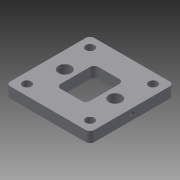
# Autodesk Inventor part: AdapterPlate
Saved by Autodesk Inventor 2015 SP1 (Build 190203100, 203)
## iProperties
Created: 2015-08-27
Part Number: AdapterPlate
Material: Generic
Document SubType Name: Modeling
Designer: I Rabey
Density: 1 g/cm^3
Appearance: Default
Author: I Rabey
Autodesk Inventor part; units mm, degrees
ref_plane "YZ Plane" through (0, 0, 0) normal (1, 0, 0) x (0, 1, 0)
ref_plane "XZ Plane" through (0, 0, 0) normal (0, 1, 0) x (-1, 0, 0)
ref_plane "XY Plane" through (0, 0, 0) normal (0, 0, 1) x (1, 0, 0)
sketch "Sketch1" plane through (0, 0, 0) normal (0, 1, 0) x (-1, 0, 0)
  line L0 (-17.5, -17.5) -> (17.5, 17.5) construction
  line L1 (17.5, -17.5) -> (-17.5, 17.5) construction
  circle A0 centre (15, -15) radius 2.05
  circle A1 centre (-15, -15) radius 2.05
  circle A2 centre (-15, 15) radius 2.05
  circle A3 centre (15, 15) radius 2.05
  line L2 (20, 20) -> (-20, 20)
  line L3 (-20, 20) -> (-20, -20)
  line L4 (-20, -20) -> (20, -20)
  line L5 (20, -20) -> (20, 20)
  line L6 (20, 20) -> (-20, -20) construction
  line L7 (-20, 20) -> (20, -20) construction
  circle A4 centre (12, 0) radius 3.05
  circle A5 centre (-12, 0) radius 3.05
  point P0 (0, 0)
  dimension "d0" = 35
  dimension "d1" = 35
  dimension "d2" = 4.1
  dimension "d3" = 4.1
  dimension "d4" = 4.1
  dimension "d5" = 4.1
  dimension "d6" = 30
  dimension "d7" = 30
  dimension "d8" = 30
  dimension "d9" = 30
  dimension "d10" = 40
  dimension "d11" = 40
  dimension "d14" = 6.1
  dimension "d15" = 8
  dimension "d16" = 6.1
  dimension "d17" = 8
  constraints: 16 end point, 6 centre point, 4 midpoint, 4 point on line, 2 parallel, 1 horizontal, 1 perpendicular
  measures "d0" distance of L1.end L0.end
  measures "d1" distance of L1.start L0.end
  measures "d2" diameter of A0
  measures "d3" diameter of A1
  measures "d4" diameter of A2
  measures "d5" diameter of A3
  measures "d6" distance of A3.centre A0.centre
  measures "d7" distance of A0.centre A1.centre
  measures "d8" distance of A2.centre A1.centre
  measures "d9" distance of A3.centre A2.centre
  measures "d10" distance of L4.end L3.end
  measures "d11" distance of L3.end L2.end
  measures "d14" diameter of A4
  measures "d15" distance from line of A4.centre L5
  measures "d16" diameter of A5
  measures "d17" distance from line of L3 A5.centre
extrude "Extrusion2" add sketch "Sketch1" along normal blind 5
sketch "Sketch2" plane through (20, 0, 20) normal (1, 0, 0) x (0, 0, -1)
  circle A0 centre (20, 2.5) radius 1
  line L0 (0, 5) -> (40, 5) projected
  point P0 (20, 0)
  dimension "d20" = 2
  dimension "d21" = 2.5
  constraints: 1 centre point
  measures "d20" diameter of A0
  measures "d21" distance from line of A0.centre L0
hole "Hole1" at (20, 2.5, 0) direction (-1, 0, 0) diameter 2 depth 8 tip angle 118
thread "Thread1" size "M2x0.4" class "6H" standard "ANSI Metric M Profile" full length
sketch "Sketch3" plane through (-20, 0, -20) normal (-1, 0, 0) x (0, 0, 1)
  circle A0 centre (20, 2.5) radius 1 projected
  circle A1 centre (20, 2.5) radius 1
  point P0 (20, 0)
  dimension "d31" = 2
  constraints: 1 centre point, 1 coincident
  measures "d31" diameter of A1
hole "Hole2" at (-20, 2.5, 0) direction (1, 0, 0) diameter 2 depth 8 tip angle 118
thread "Thread2" size "M2x0.4" class "6H" standard "ANSI Metric M Profile" full length
sketch "Sketch4" plane through (0, 5, 0) normal (0, 1, 0) x (1, 0, 0)
  line L0 (7, -9) -> (-7, -9)
  line L1 (-7, -9) -> (-7, 9)
  line L2 (-7, 9) -> (7, 9)
  line L3 (7, 9) -> (7, -9)
  line L4 (7, -9) -> (-7, 9) construction
  line L5 (-7, -9) -> (7, 9) construction
  point P0 (0, 0)
  dimension "d41" = 14
  dimension "d42" = 18
  constraints: 12 end point, 2 midpoint, 2 parallel, 1 horizontal, 1 perpendicular
  measures "d41" distance of L1.end L2.end
  measures "d42" distance of L0.end L1.end
extrude "Extrusion3" cut sketch "Sketch4" against normal blind 10
fillet "Fillet1" radius 2 1 edges at (20, 2.5, 20)
fillet "Fillet2" radius 2 1 edges at (20, 2.5, -20)
fillet "Fillet3" radius 2 1 edges at (-20, 2.5, -20)
fillet "Fillet4" radius 2 1 edges at (-20, 2.5, 20)
fillet "Fillet5" radius 2 1 edges at (-7, 2.5, -9)
fillet "Fillet6" radius 2 1 edges at (-7, 2.5, 9)
fillet "Fillet7" radius 2 1 edges at (7, 2.5, -9)
fillet "Fillet8" radius 2 1 edges at (7, 2.5, 9)
body "Solid2"
